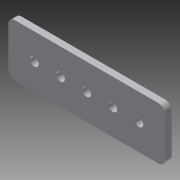
# Autodesk Inventor part: 3 X 1 Spacer
Saved by Autodesk Inventor 2014 (Build 180170000, 170)
## iProperties
Created: 2014-01-07
Part Number: 3 X 1 Spacer
Material: Aluminum 6061
Document SubType Name: Modeling
Designer: Michael
Density: 2.71 g/cm^3
Appearance: Aluminum - Flat
Author: Michael
Autodesk Inventor part; units mm, degrees
ref_plane "YZ Plane" through (0, 0, 0) normal (1, 0, 0) x (0, 1, 0)
ref_plane "XZ Plane" through (0, 0, 0) normal (0, 1, 0) x (-1, 0, 0)
ref_plane "XY Plane" through (0, 0, 0) normal (0, 0, 1) x (1, 0, 0)
sketch "Sketch1" plane through (0, 0, 0) normal (0, 0, 1) x (1, 0, 0)
  line L0 (0, 0) -> (76.2, 0)
  line L1 (76.2, 0) -> (76.2, 25.4)
  line L2 (76.2, 25.4) -> (0, 25.4)
  line L3 (0, 25.4) -> (0, 0)
  circle A0 centre (12.7, 12.7) radius 2.0828
  circle A1 centre (25.4, 12.7) radius 2.0828
  circle A2 centre (38.1, 12.7) radius 2.0828
  circle A3 centre (50.8, 12.7) radius 2.0828
  circle A4 centre (63.5, 12.7) radius 2.0828
  dimension "d0" = 76.2
  dimension "d1" = 25.4
  dimension "d2" = 4.1656
  dimension "d3" = 12.7
  dimension "d4" = 12.7
  dimension "d7" = 12.7
  constraints: 8 end point, 5 centre point, 2 horizontal, 2 parallel, 1 perpendicular, 8 other
  measures "d0" distance of L2.end L1.end
  measures "d1" distance of L1.end L0.end
  measures "d2" diameter of A0
  measures "d3" distance from line of L0 A0.centre
  measures "d4" distance from line of L3 A0.centre
  measures "d7" distance of A0.centre A1.centre
extrude "Extrusion1" add sketch "Sketch1" along normal blind 3.175
fillet "Fillet1" radius 3.175 4 edges at (0, 25.4, 1.5875) (0, 0, 1.5875) (76.2, 0, 1.5875) (76.2, 25.4, 1.5875)
body "Solid1"
